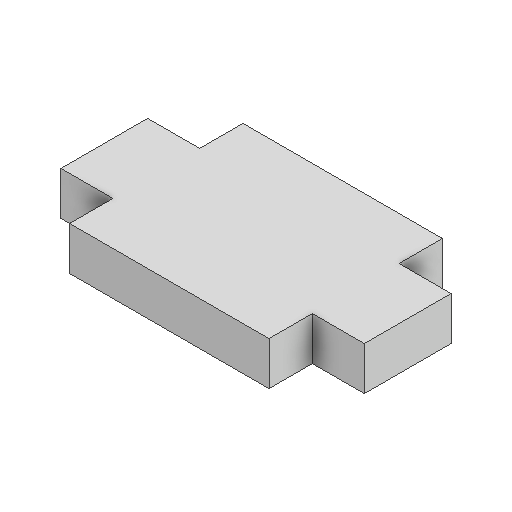
# Autodesk Inventor part: Подставка для двигателя и драйвера
Saved by Autodesk Inventor 2022 (Build 260153000, 153)
## iProperties
Created: 2023-02-18
Part Number: Подставка для двигателя и драйвера
Material: Типовые
Document SubType Name: Modeling
Designer: Глеб
Density: 1 g/cm^3
Appearance: По умолчанию
Author: Глеб
Autodesk Inventor part; units mm, degrees
ref_plane "YZ Plane" through (0, 0, 0) normal (1, 0, 0) x (0, 1, 0)
ref_plane "XZ Plane" through (0, 0, 0) normal (0, 1, 0) x (-1, 0, 0)
ref_plane "XY Plane" through (0, 0, 0) normal (0, 0, 1) x (1, 0, 0)
sketch "Эскиз1" plane through (0, 0, 0) normal (1, 0, 0) x (0, 1, 0)
  line L0 (-5, 10) -> (5, 10)
  line L1 (5, 10) -> (5, -10)
  line L2 (5, -10) -> (-5, -10)
  line L3 (-5, -10) -> (-5, 10)
  line L4 (-5, 10) -> (5, -10) construction
  line L5 (5, 10) -> (-5, -10) construction
  point P0 (0, 0)
  dimension "d0" = 10
  dimension "d1" = 20
  constraints: 12 end point, 2 midpoint, 2 parallel, 1 horizontal, 1 perpendicular
  measures "d0" distance between parallel lines of L3 L1
  measures "d1" distance between parallel lines of L2 L0
extrude "Выдавливание1" add sketch "Эскиз1" along normal mid plane 70
sketch "Эскиз2" plane through (-35, 5, 10) normal (0, 1, 0) x (1, 0, 0)
  line L0 (58, -42.6795) -> (58, 140) construction
  line L1 (70, 140) -> (70, -60) construction
  line L2 (0, 20) -> (70, 20) construction
  line L3 (0, 0) -> (70, 0) construction
  line L4 (58, 20) -> (12, 20)
  line L5 (12, 20) -> (12, 30)
  line L6 (12, 30) -> (58, 30)
  line L7 (58, 30) -> (58, 20)
  line L8 (0, 0) -> (0, 20) projected
  line L9 (58, 0) -> (12, 0)
  line L10 (12, 0) -> (12, -10)
  line L11 (12, -10) -> (58, -10)
  line L12 (58, -10) -> (58, 0)
  dimension "d27" = 10
  dimension "d28" = 10
  dimension "d30" = 12
  dimension "d31" = 46
  dimension "d32" = 46
  dimension "d33" = 12
  constraints: 16 end point, 4 parallel, 2 horizontal, 2 perpendicular, 2 point on line
  measures "d27" distance of L4.end L5.end
  measures "d28" distance of L9.end L10.end
  measures "d30" distance between parallel lines of L8 L10
  measures "d31" distance of L5.end L6.end
  measures "d32" distance of L10.end L11.end
  measures "d33" distance between parallel lines of L1 L7
extrude "Выдавливание2" add sketch "Эскиз2" against normal blind 10
equation "\"d28\" = d27"
equation "\"d30\" = d26"
equation "\"d32\" = d31"
equation "\"d26\" = d25"
equation "\"d25\" = 12"
